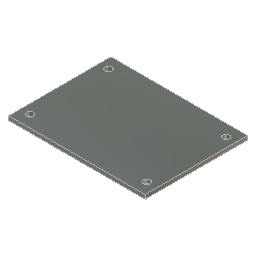
ST7889_240x240_Display (Autodesk Fusion 360 design; units mm, degrees)
Autodesk Fusion 360 part; units mm, degrees
sketch "Sketch1" plane through (0, 0, 0) normal (0, 0, 1) x (1, 0, 0)
  line L0 (0, 0) -> (40, 0)
  line L1 (40, 0) -> (40, 30)
  line L2 (40, 30) -> (0, 30)
  line L3 (0, 30) -> (0, 0)
  dimension "d1" = 40
  dimension "d2" = 30
  constraint horizontal L0
  constraint vertical L1
  constraint horizontal L2
  constraint vertical L3
  constraint coincident L0.start L3.end
  measures "d1" distance of L0.start L0.end
  measures "d2" distance of L0.start L2.end
extrude "Extrude1" add sketch "Sketch1" along normal blind 1.2
sketch "Sketch2" plane through (0, 0, 1.2) normal (0, 0, 1) x (-1, 0, 0)
  line L0 (0, -30) -> (0, 0)
  line L1 (0, 0) -> (-40, 0)
  line L2 (-40, 0) -> (-40, -30)
  line L3 (-40, -30) -> (0, -30)
sketch "Sketch3" plane through (0, 0, 1.2) normal (0, 0, 1) x (-1, 0, 0)
sketch "Sketch4" plane through (0, 0, 1.2) normal (0, 0, 1) x (-1, 0, 0)
  line L0 (-40, 0) -> (-40, -30)
  line L1 (-40, -30) -> (0, -30)
  circle A0 centre (-2.75, -26.5) radius 1
  circle A1 centre (-2.75, -3.5) radius 1
  circle A2 centre (-37.25, -26.5) radius 1
  circle A3 centre (-37.0314, -3.5) radius 1
  point P0 (-20, -30)
  point P1 (-40, -15)
  point P2 (-37.25, -26.5)
  point P3 (-37.0314, -3.5)
  point P4 (-2.75, -26.5)
  point P5 (-2.75, -3.5)
  dimension "d8" = 11.5
  dimension "d9" = 17.25
  dimension "d10" = 23
  dimension "d11" = 34.5
  dimension "d12" = 2
  dimension "d13" = 2
  dimension "d14" = 2
  dimension "d15" = 2
  constraint midpoint P0 L1
  constraint midpoint L0 P1
  constraint horizontal P2 P4
  constraint vertical P4 P5
  constraint horizontal P3 P5
  constraint coincident P4 A0.centre
  constraint coincident P5 A1.centre
  constraint coincident P2 A2.centre
  constraint coincident P3 A3.centre
  measures "d8" vertical distance of P1 P2
  measures "d9" horizontal distance of P0 P2
  measures "d10" vertical distance of P2 P3
  measures "d11" horizontal distance of P2 P4
  measures "d12" diameter of A0
  measures "d13" diameter of A1
  measures "d14" diameter of A2
  measures "d15" diameter of A3
hole "Hole1" at (2.75, 3.5, 1.2) at (37.0314, 3.5, 1.2) at (37.25, 26.5, 1.2) at (2.75, 26.5, 1.2) direction (0, 0, -1) diameter 2 depth 1.5 tip angle 180
